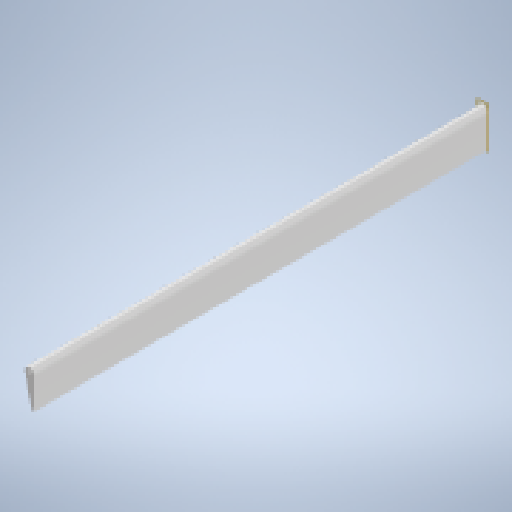
# Autodesk Inventor part: AlerionLeft
Saved by Autodesk Inventor 2026 (Build 300175050, 175E)
## iProperties
Created: 2025-08-01
Part Number: AlerionLeft
Material: Generic
Document SubType Name: Modeling
Designer: Cupri
Density: 1 g/cm^3
Appearance: Default
Author: Cupri
Autodesk Inventor part; units mm, degrees
ref_plane "YZ Plane" through (0, 0, 0) normal (1, 0, 0) x (0, 1, 0)
ref_plane "XZ Plane" through (0, 0, 0) normal (0, 1, 0) x (-1, 0, 0)
ref_plane "XY Plane" through (0, 0, 0) normal (0, 0, 1) x (1, 0, 0)
ref_plane "Work Plane1" through (0, 0, 0) normal (0, 0, 1) x (1, 0, 0)
sketch "Sketch1" plane through (0, 0, 0) normal (0, 0, 1) x (1, 0, 0)
  circle A0 centre (-5.0231, -8) radius 1.5
  spline S0 degree 3 poles (0.9769, 0) (0.942164, -1.701599) (0.907899, -3.46781) (0.874191, -5.266511) knots 0.0501942 0.0501942 0.0501942 0.0501942 0.55684644 0.55684644 0.55684644 0.55684644
  arc A1 (0.874191, -5.266511) -> (-11.114321, -5.731295) centre (-5.0231, -8) ccw
  spline S1 degree 3 poles (-11.114321, -5.731295) (-11.524724, -3.794172) (-11.922878, -1.876516) (-12.304521, 0) knots 4.69387335 4.69387335 4.69387335 4.69387335 5.24003316 5.24003316 5.24003316 5.24003316
  line L0 (-12.304521, 0) -> (-12.307312, 0)
  line L1 (-12.307312, 0) -> (-12.919596, 0)
  spline S2 degree 3 poles (-0.911816, -50) (-3.27117, -41.164888) (-4.436234, -37.226907) (-8.629504, -20.079006) (-10.989776, -9.492834) (-12.919596, 0) knots -5.64844745 -5.64844745 -5.64844745 -5.64844745 -2.94452824 -2.94452824 -0.05090828 -0.05090828 -0.05090828 -0.05090828
  line L2 (-0.341845, -49.847793) -> (-0.911816, -50)
  line L3 (-0.341845, -49.847793) -> (0.75, -49.847793)
  line L4 (0.75, -49.847006) -> (0.75, -49.847793)
  line L5 (0.932124, -49.847793) -> (0.75, -49.847006)
  spline S3 degree 3 poles (1.530662, -2.317659) (1.356238, -11.22636) (1.198334, -21.474255) (0.99681, -36.986495) (0.969082, -41.30095) (0.932124, -49.847793) knots -4.87507574 -4.87507574 -4.87507574 -4.87507574 -2.56407697 -2.56407697 0 0 0 0
  spline S4 degree 3 poles (1.576974, 0) (1.561468, -0.760263) (1.54601, -1.533777) (1.530662, -2.317659) knots 0 0 0 0 1 1 1 1
  line L6 (1.576974, 0) -> (0.9769, 0)
  line L7 (-11.114321, -5.731295) -> (-11.506873, -6.785252)
  line L8 (0.874191, -5.266511) -> (1.446469, -6.785252)
  line L9 (0.932124, -49.847793) -> (0.932124, -50)
  line L10 (0.932124, -50) -> (-0.911816, -50)
  arc A2 (1.26114, -7.554657) -> (-11.315142, -7.683447) centre (-5.0231, -8) ccw
  line L11 (1.215655, -7.123677) -> (1.40786, -8.944856)
  point P0 (0, 0)
  dimension "d2" = 0.2
  constraints: 10 end point, 3 point on circle, 1 centre point, 1 coincident, 1 perpendicular, 1 point on line, 1 tangent, 1 vertical, 4 other
  measures "d2" radial gap between concentric circles of A1 A2
ref_plane "Work Plane2" through (-13.55541, -50.053146, 600) normal (0, 0, -1) x (0, 1, 0)
extrude "Extrusion1" add sketch "Sketch1" along normal up to surface (600 mm away) contours S3 L5 L3 L2 S2 A2 L11 | L9 L10 L2 L3 L5 | L11 A2
body "Solid1"
